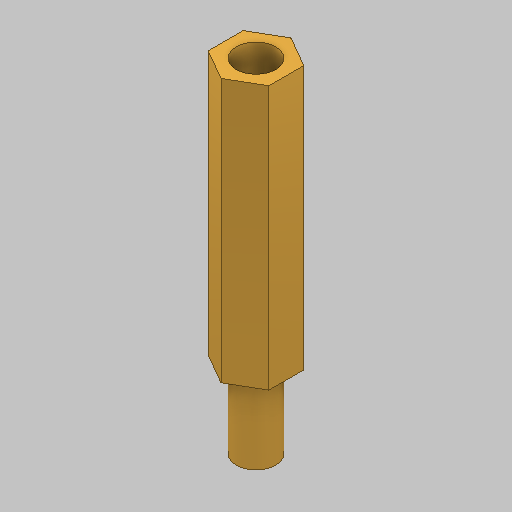
# Autodesk Inventor part: Separador-M3-20mm-Pin
Saved by Autodesk Inventor 2024.2 (Build 282272000, 272)
## iProperties
Created: 2023-09-25
Part Number: Separador-M3-20mm-Pin
Material: Stainless Steel
Document SubType Name: Modeling
Designer: jalva
Density: 8 g/cm^3
Appearance: Brass - Satin
Mass: 2.42308 g
Surface Area: 5.53268 cm^2
Volume: 0.302885 cm^3
Author: jalva
Autodesk Inventor part; units mm, degrees
ref_plane "YZ Plane" through (0, 0, 0) normal (1, 0, 0) x (0, 1, 0)
ref_plane "XZ Plane" through (0, 0, 0) normal (0, 1, 0) x (-1, 0, 0)
ref_plane "XY Plane" through (0, 0, 0) normal (0, 0, 1) x (1, 0, 0)
sketch "Sketch1" plane through (0, 0, 0) normal (0, 1, 0) x (-1, 0, 0)
  line L0 (0, -2.6558) -> (-2.3, -1.3279)
  line L1 (-2.3, -1.3279) -> (-2.3, 1.3279)
  line L2 (-2.3, 1.3279) -> (0, 2.6558)
  line L3 (0, 2.6558) -> (2.3, 1.3279)
  line L4 (2.3, 1.3279) -> (2.3, -1.3279)
  line L5 (2.3, -1.3279) -> (0, -2.6558)
  point P0 (0, 0)
  point P1 (0, 0)
  dimension "d0" = 4.6
  constraints: 12 end point, 1 coincident, 1 vertical, 13 other
  measures "d0" distance between parallel lines of L1 L4
extrude "Extrusion1" add sketch "Sketch1" along normal blind 20
sketch "Sketch2" plane through (0, 20, 0) normal (0, 1, 0) x (1, 0, 0)
  circle A0 centre (0, 0) radius 1.5
  dimension "d3" = 3
  constraints: 1 centre point, 1 coincident
  measures "d3" diameter of A0
extrude "Extrusion2" cut sketch "Sketch2" against normal blind 15
sketch "Sketch3" plane through (0, 0, 0) normal (0, -1, 0) x (1, 0, 0)
  circle A0 centre (0, 0) radius 1.5
  dimension "d6" = 3
  constraints: 1 centre point, 1 coincident
  measures "d6" diameter of A0
extrude "Extrusion3" add sketch "Sketch3" along normal blind 6
body "Solid1"
